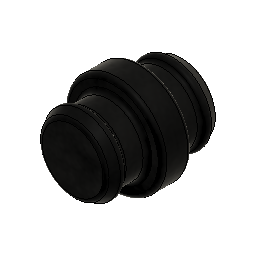
20021-013_landing-gear-foot (Autodesk Fusion 360 design; units mm, degrees)
Autodesk Fusion 360 part; units mm, degrees
sketch "Sketch1" plane through (0, 0, 0) normal (1, 0, 0) x (0, 1, 0)
  line L0 (0, 0) -> (0, 6.1)
  line L1 (0, 6.1) -> (2.97, 7.7)
  line L2 (2.97, 7.7) -> (2.97, 6.34)
  line L3 (2.97, 6.34) -> (7.5, 6.34)
  line L4 (7.5, 6.34) -> (7.5, 9.14)
  line L5 (7.5, 9.14) -> (13, 9.14)
  line L6 (13, 9.14) -> (13, 6.34)
  line L7 (13, 6.34) -> (17.53, 6.34)
  line L8 (17.53, 6.34) -> (17.53, 7.7)
  line L9 (17.53, 7.7) -> (20.5, 6.1)
  line L10 (20.5, 6.1) -> (20.5, 0)
  line L11 (20.5, 0) -> (0, 0)
  line L12 (0, 5) -> (20.5, 5)
  line L13 (1.2, 5) -> (1.2, 0)
  dimension "d1" = 7.7
  dimension "d2" = 6.34
  dimension "d3" = 5
  dimension "d4" = 6.1
  dimension "d5" = 9.14
  dimension "d6" = 20.5
  dimension "d7" = 5.5
  dimension "d8" = 4.53
  dimension "d9" = 1.2
  constraint coincident L0.start L11.end
  constraint vertical L0
  constraint parallel L0 L2
  constraint perpendicular L0 L3
  constraint perpendicular L3 L4
  constraint perpendicular L0 L5
  constraint perpendicular L5 L6
  constraint perpendicular L0 L7
  constraint perpendicular L7 L8
  constraint parallel L6 L10
  constraint perpendicular L10 L11
  constraint coincident L0 L12.start
  constraint coincident L10 L12.end
  constraint perpendicular L10 L12
  constraint equal L4 L6
  constraint equal L3 L7
  constraint equal L2 L8
  constraint equal L1 L9
  constraint horizontal L0.end L9.end
  constraint coincident L12 L13.start
  constraint coincident L11 L13.end
  constraint perpendicular L11 L13
  measures "d1" distance of L1.end L11
  measures "d2" distance of L3 L11
  measures "d3" distance of L11 L12
  measures "d4" distance of L0.end L11
  measures "d5" distance of L5 L11
  measures "d6" distance of L0 L10
  measures "d7" distance of L4.end L5.end
  measures "d8" distance of L2 L4
  measures "d9" distance of L0 L13
revolve "Revolve1" add sketch "Sketch1" angle 360 about axis through (0, 20.5, 0) along (0, -1, 0) contours L0 L11 L12 L13 | L0 L1 L2 L3 L4 L5 L6 L7 L8 L9 L10 L12
fillet "Fillet1" radius 0.8 13 faces at (0.6313, 16.02, 6.3085) (0.7691, 13, 8.149) (0.4541, 7.5, 8.1726) (0.4556, 11.1667, 9.1286) (4.8746, 1.98, 5.2535) (0.6313, 5.99, 6.3085) (0.3825, 2.97, 7.218) (0.3031, 0, 5.7106) (1.9935, 1.2, 1.3101) (0.3825, 17.53, 7.218) (6.6713, 18.52, -2.6183) (0.3031, 20.5, 5.7106) (0.4978, 7.6333, 4.9752)
equation "d1 = ( 15.4 / 2 ) * 1 mm"
equation "d2 = ( 12.68 / 2 ) * 1 mm"
equation "d4 = ( 12.2 / 2 ) * 1 mm"
equation "d5 = 18.28 mm / 2"
named bodies: "20021-013_landing-gear-foot"
